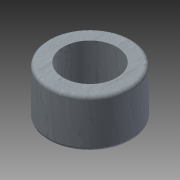
# Autodesk Inventor part: MotorWheel
Saved by Autodesk Inventor 2014 SP1 (Build 180222100, 222)
## iProperties
Created: 2015-03-22
Part Number: MotorWheel
Material: Generic
Document SubType Name: Modeling
Designer: david
Density: 1 g/cm^3
Appearance: Default
Author: david
Autodesk Inventor part; units mm, degrees
ref_plane "YZ Plane" through (0, 0, 0) normal (1, 0, 0) x (0, 1, 0)
ref_plane "XZ Plane" through (0, 0, 0) normal (0, 1, 0) x (-1, 0, 0)
ref_plane "XY Plane" through (0, 0, 0) normal (0, 0, 1) x (1, 0, 0)
sketch "Sketch1" plane through (0, 0, 0) normal (0, 1, 0) x (-1, 0, 0)
  circle A0 centre (0, 0) radius 15
  circle A1 centre (0, 0) radius 23.5
  dimension "d0" = 30
  dimension "d1" = 47
  constraints: 2 centre point, 2 coincident
  measures "d0" diameter of A0
  measures "d1" diameter of A1
extrude "Extrusion1" add sketch "Sketch1" along normal blind 27
fillet "Fillet1" radius 2 2 edges at (23.5, 27, 0) (23.5, 0, 0)
equation "\"d0\" = Motor_WheelInterface_Diameter"
equation "\"d1\" = MotorWheel_Diameter"
equation "\"d2\" = MotorWheel_Width"
equation "\"MotorWheel_Diameter\" = 47"
equation "\"MotorWheel_Width\" = Motor_WheelInterface_Length"
equation "\"Motor_WheelInterface_Diameter\" = 30"
equation "\"Motor_WheelInterface_Length\" = 27"
body "Solid1"
